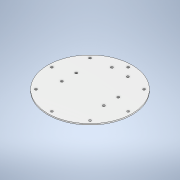
# Autodesk Inventor part: pcbCase_last
Saved by Autodesk Inventor 2020 (Build 240168000, 168)
## iProperties
Created: 2020-04-07
Part Number: pcbCase_last
Material: Пластик АБС
Document SubType Name: Modeling
Designer: jamnissa
Density: 1.06 g/cm^3
Appearance: Гладкий — белый
Mass: 15.0891 g
Surface Area: 195.671 cm^2
Volume: 15.0891 cm^3
Author: jamnissa
Autodesk Inventor part; units mm, degrees
ref_plane "YZ Plane" through (0, 0, 0) normal (1, 0, 0) x (0, 1, 0)
ref_plane "XZ Plane" through (0, 0, 0) normal (0, 1, 0) x (-1, 0, 0)
ref_plane "XY Plane" through (0, 0, 0) normal (0, 0, 1) x (1, 0, 0)
sketch "Эскиз1" plane through (0, 0, 0) normal (0, 1, 0) x (-1, 0, 0)
  circle A0 centre (0, 0) radius 55
  line L0 (79.4555, 0) -> (-79.4555, 0)
  line L1 (0, -103.8803) -> (0, 88.3129)
  line L2 (38.15, -21.1) -> (-38.15, -21.1)
  line L3 (-38.15, -21.1) -> (-38.15, 21.1)
  line L4 (-38.15, 21.1) -> (38.15, 21.1)
  line L5 (38.15, 21.1) -> (38.15, -21.1)
  dimension "d0" = 110
  dimension "d60" = 76.3
  dimension "d61" = 42.2
  constraints: 12 end point, 2 horizontal, 2 parallel, 1 centre point, 1 coincident, 1 midpoint, 1 perpendicular, 1 point on line, 1 vertical, 2 other
  measures "d0" diameter of A0
  measures "d60" distance of L3.end L4.end
  measures "d61" distance of L4.end L2.start
extrude "Выдавливание1" add sketch "Эскиз1" along normal blind 1.6
sketch "Эскиз2" plane through (0, 0, 0) normal (0, -1, 0) x (1, 0, 0)
  circle A0 centre (0, 0) radius 55 projected
  line L0 (0, -103.8803) -> (0, 88.3129)
  line L1 (-79.4555, 0) -> (79.4555, 0) projected
  circle A1 centre (0, 0) radius 50
  circle A2 centre (0, -50) radius 1.5
  circle A3 centre (50, 0) radius 1.5
  circle A4 centre (0, 50) radius 1.5
  circle A5 centre (-50, 0) radius 1.5
  circle A6 centre (35.3553, -35.3553) radius 1.5
  circle A7 centre (50, 0) radius 1.5
  circle A8 centre (35.3553, 35.3553) radius 1.5
  circle A9 centre (0, 50) radius 1.5
  circle A10 centre (-35.3553, 35.3553) radius 1.5
  circle A11 centre (-50, 0) radius 1.5
  circle A12 centre (-35.3553, -35.3553) radius 1.5
  line L2 (38.15, -20) -> (-39.85, -20)
  line L3 (-39.85, -20) -> (-39.85, 20)
  line L4 (-39.85, 20) -> (38.15, 20)
  line L5 (38.15, 20) -> (38.15, -20)
  line L6 (-27.5, 9.5) -> (27.5, 9.5)
  line L7 (27.5, 9.5) -> (27.5, -9.5)
  line L8 (27.5, -9.5) -> (-27.5, -9.5)
  line L9 (-27.5, -9.5) -> (-27.5, 9.5)
  circle A13 centre (27.5, 9.5) radius 1.5
  circle A14 centre (-27.5, 9.5) radius 1.5
  circle A15 centre (-27.5, -9.5) radius 1.5
  circle A16 centre (27.5, -9.5) radius 1.5
  circle A17 centre (0, -50) radius 1.5
  circle A18 centre (-10.5, -39) radius 1.5
  circle A19 centre (10.5, -39) radius 1.5
  point P0 (11.9394, -0.2)
  dimension "d22" = 3
  dimension "d23" = 3
  dimension "d25" = 3
  dimension "d26" = 3
  dimension "d30" = 360
  dimension "d62" = 78
  dimension "d63" = 40
  dimension "d70" = 110
  dimension "d71" = 55
  dimension "d72" = 19
  dimension "d73" = 3
  dimension "d74" = 3
  dimension "d75" = 3
  dimension "d76" = 3
  constraints: 19 centre point, 18 end point, 5 coincident, 4 parallel, 4 point on circle, 4 point on line, 2 horizontal, 2 perpendicular, 20 other
  measures "d22" diameter of A2
  measures "d23" diameter of A3
  measures "d25" diameter of A4
  measures "d26" diameter of A5
  measures "d62" distance of L3.end L4.end
  measures "d63" distance of L4.end L2.start
  measures "d70" diameter of A0
  measures "d71" distance of L6.start L6.end
  measures "d72" distance of L6.end L7.end
  measures "d73" diameter of A13
  measures "d74" diameter of A14
  measures "d75" diameter of A15
  measures "d76" diameter of A16
extrude "Выдавливание2" cut sketch "Эскиз2" against normal blind 1.6 contours A3 A1 L1 | L1 A1 A3 | A4 A1 L0 | L0 A1 A4 | A2 A1 L0 | L0 A1 A2 | A1 A3 L1 | L1 A3 A1 | A5 A1 L1 | L1 A1 A5 | A1 A4 L0 | L0 A4 A1 | A1 A2 L0 | L0 A2 A1 | A8 A1 | A1 A8 | A6 A1 | A1 A6 | A1 A5 L1 | L1 A5 A1 | A10 A1 | A1 A10 | A12 A1 | A1 A12
extrude "Выдавливание5" [suppressed]
extrude "Выдавливание6" cut sketch "Эскиз2" against normal blind 10 contours A13 L6 L7 | L7 L6 A13 | A16 L8 L7 | L7 L8 A16 | A14 L9 L6 | L6 L9 A14 | A15 L9 L8 | L8 L9 A15 | A18 | A19
